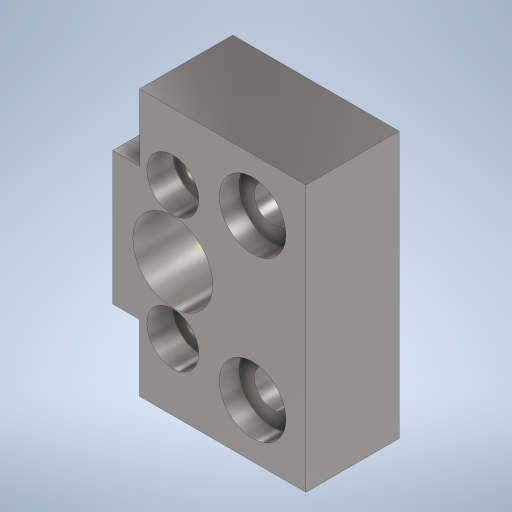
# Autodesk Inventor part: MotorMount
Saved by Autodesk Inventor 2023 (Build 270158000, 158)
## iProperties
Created: 2023-03-27
Part Number: MotorMount
Material: Stainless Steel
Document SubType Name: Modeling
Designer: Nathann
Density: 8 g/cm^3
Appearance: Semi-Polished
Mass: 11.2507 g
Surface Area: 13.5845 cm^2
Volume: 1.40634 cm^3
Author: Nathann
Autodesk Inventor part; units mm, degrees
ref_plane "YZ Plane" through (0, 0, 0) normal (1, 0, 0) x (0, 1, 0)
ref_plane "XZ Plane" through (0, 0, 0) normal (0, 1, 0) x (-1, 0, 0)
ref_plane "XY Plane" through (0, 0, 0) normal (0, 0, 1) x (1, 0, 0)
sketch "Sketch1" plane through (0, 0, 0) normal (0, 0, 1) x (1, 0, 0)
  line L0 (10, -10) -> (-10, -10)
  line L1 (-10, -10) -> (-10, 10)
  line L2 (-10, 10) -> (10, 10)
  line L3 (10, 10) -> (10, -10)
  circle A0 centre (0, 5) radius 1.2
  circle A1 centre (0, -5) radius 1.2
  circle A2 centre (0, 0) radius 3
  dimension "d0" = 10
  dimension "d1" = 10
  dimension "d2" = 10
  dimension "d3" = 10
  dimension "d4" = 5
  dimension "d5" = 5
  dimension "d6" = 2.4
  dimension "d7" = 2.4
  dimension "d8" = 6
  constraints: 8 end point, 3 centre point, 2 parallel, 1 coincident, 1 horizontal, 1 perpendicular
  measures "d0" distance from line of L1 point (0, 0)
  measures "d1" distance from line of L3 point (0, 0)
  measures "d2" distance from line of L0 point (0, 0)
  measures "d3" distance from line of L2 point (0, 0)
  measures "d4" distance of point (0, 0) A0.centre
  measures "d5" distance of point (0, 0) A1.centre
  measures "d6" diameter of A0
  measures "d7" diameter of A1
  measures "d8" diameter of A2
extrude "Extrusion1" add sketch "Sketch1" along normal blind 5
sketch "Sketch2" plane through (0, 0, 5) normal (0, 0, 1) x (1, 0, 0)
  line L0 (0, 0) -> (-1.3346, -1.3533)
  circle A0 centre (6, -6) radius 2.5
  circle A1 centre (6, 6) radius 2.5
  line L1 (10, -10) -> (10, 10) projected
  line L2 (-10, -10) -> (10, -10) projected
  line L3 (10, 10) -> (-10, 10) projected
  dimension "d34" = 4
  dimension "d35" = 4
  dimension "d36" = 4
  dimension "d37" = 4
  dimension "d38" = 5
  dimension "d39" = 5
  constraints: 2 centre point, 2 end point, 1 other
  measures "d34" distance from line of L1 A0.centre
  measures "d35" distance from line of L2 A0.centre
  measures "d36" distance from line of L3 A1.centre
  measures "d37" distance from line of L1 A1.centre
  measures "d38" diameter of A1
  measures "d39" diameter of A0
extrude "Extrusion2" cut sketch "Sketch2" against normal blind 1
sketch "Sketch7" plane through (0, 0, 0) normal (0, 0, -1) x (-1, 0, 0)
  circle A0 centre (-6, 6) radius 2.5 projected
  circle A1 centre (-6, 6) radius 1.375
  circle A2 centre (-6, -6) radius 2.5 projected
  circle A3 centre (-6, -6) radius 1.375
  point P0 (0, 0)
  dimension "d40" = 2.75
  dimension "d41" = 2.75
  constraints: 2 centre point, 2 coincident
  measures "d40" diameter of A1
  measures "d41" diameter of A3
extrude "Extrusion6" cut sketch "Sketch7" against normal blind 5 contours A1 | A3
sketch "Sketch8" plane through (0, 0, 5) normal (0, 0, 1) x (1, 0, 0)
  line L0 (10, 10) -> (-10, 10) projected
  line L1 (10, 10) -> (2.5, 10)
  line L2 (2.5, 10) -> (2.5, 2.5)
  line L3 (2.5, 2.5) -> (10, 2.5)
  line L4 (10, 2.5) -> (10, 10)
  line L5 (10, -10) -> (10, 10) projected
  line L6 (10, -10) -> (2.5, -10)
  line L7 (2.5, -10) -> (2.5, -2.5)
  line L8 (2.5, -2.5) -> (10, -2.5)
  line L9 (10, -2.5) -> (10, -10)
  line L10 (10, -2.5) -> (5, -2.5)
  line L11 (5, -2.5) -> (5, 2.5)
  line L12 (5, 2.5) -> (10, 2.5)
  line L13 (10, 2.5) -> (10, -2.5)
  circle A0 centre (6, 6) radius 2.5 projected
  circle A1 centre (6, 6) radius 2.5
  circle A2 centre (6, -6) radius 2.5 projected
  circle A3 centre (6, -6) radius 2.5
  point P0 (0, 0)
  point P1 (2.5, 10)
  dimension "d44" = 7.5
  dimension "d45" = 7.5
  dimension "d46" = 7.5
  dimension "d47" = 7.5
  dimension "d48" = 5
  constraints: 24 end point, 6 parallel, 3 horizontal, 3 perpendicular, 2 centre point, 2 coincident, 2 point on line
  measures "d44" distance between parallel lines of L4 L2
  measures "d45" distance of L1.end L2.end
  measures "d46" distance of L6.end L7.end
  measures "d47" distance of L5.start L6.end
  measures "d48" distance between parallel lines of L5 L11
extrude "Extrusion7" add sketch "Sketch8" along normal blind 2
sketch "Sketch9" plane through (0, 0, 0) normal (0, 0, -1) x (-1, 0, 0)
  circle A0 centre (-6, 6) radius 1.375 projected
  circle A1 centre (-6, 6) radius 2.5
  circle A2 centre (-6, -6) radius 1.375 projected
  circle A3 centre (-6, -6) radius 2.5
  point P0 (0, 0)
  dimension "d51" = 5
  dimension "d52" = 5
  constraints: 2 centre point, 2 coincident
  measures "d51" diameter of A1
  measures "d52" diameter of A3
extrude "Extrusion8" cut sketch "Sketch9" against normal blind 2.5 contours A0 | A1 | A2 | A3
sketch "Sketch10" plane through (0, 0, 0) normal (0, 0, -1) x (-1, 0, 0)
  line L0 (-2.5, 10) -> (10, 10) projected
  line L1 (10, -10) -> (-2.5, -10) projected
  line L2 (10, 10) -> (5, 10)
  line L3 (5, 10) -> (5, -10)
  line L4 (5, -10) -> (10, -10)
  line L5 (10, -10) -> (10, 10)
  line L6 (5, 10) -> (2.5, 10)
  line L7 (2.5, 10) -> (2.5, 5)
  line L8 (2.5, 5) -> (5, 5)
  line L9 (5, 5) -> (5, 10)
  line L10 (5, -10) -> (2.5, -10)
  line L11 (2.5, -10) -> (2.5, -5)
  line L12 (2.5, -5) -> (5, -5)
  line L13 (5, -5) -> (5, -10)
  point P0 (0, 0)
  point P1 (2.5, 10)
  dimension "d55" = 5
  dimension "d56" = 2.5
  dimension "d57" = 5
  dimension "d58" = 5
  dimension "d59" = 2.5
  constraints: 24 end point, 6 parallel, 3 horizontal, 3 perpendicular, 2 point on line
  measures "d55" distance between parallel lines of L5 L3
  measures "d56" distance of L7.end L8.end
  measures "d57" distance of L6.end L7.end
  measures "d58" distance of L10.end L11.end
  measures "d59" distance of L11.end L12.end
extrude "Extrusion9" cut sketch "Sketch10" against normal blind 10
sketch "Sketch12" plane through (6, -6, 4) normal (0, 0, 1) x (1, 0, 0)
  circle A0 centre (0, 0) radius 1.375 projected
  circle A1 centre (0, 0) radius 2.5 projected
  circle A2 centre (0, 12) radius 2.5 projected
  circle A3 centre (0, 12) radius 1.375 projected
  circle A4 centre (0, 12) radius 2.5 projected
  point P0 (-6, 6)
extrude "Extrusion11" add sketch "Sketch12" along normal blind 1.5
sketch "Sketch13" plane through (0, 0, 5) normal (0, 0, 1) x (1, 0, 0)
  point P0 (0, 0)
sketch "Sketch14" plane through (0, 0, 5) normal (0, 0, 1) x (1, 0, 0)
  line L0 (-2.5, -5) -> (-2.5, -10) projected
  line L1 (-2.5, -10) -> (2.5, -10) projected
  line L2 (2.5, -10) -> (2.5, -2.5) projected
  line L3 (2.5, -2.5) -> (5, -2.5) projected
  line L4 (5, -2.5) -> (5, 2.5) projected
  line L5 (5, 2.5) -> (2.5, 2.5) projected
  line L6 (2.5, 2.5) -> (2.5, 10) projected
  line L7 (2.5, 10) -> (-2.5, 10) projected
  line L8 (-2.5, 10) -> (-2.5, 5) projected
  line L9 (-2.5, 5) -> (-5, 5) projected
  line L10 (-5, 5) -> (-5, -5) projected
  line L11 (-5, -5) -> (-2.5, -5) projected
  circle A0 centre (0, 0) radius 3 projected
  circle A1 centre (0, -5) radius 1.2 projected
  circle A2 centre (0, 5) radius 1.2 projected
  circle A3 centre (0, -5) radius 1.95
  circle A4 centre (0, 5) radius 1.95
  dimension "d80" = 3.9
  dimension "d81" = 3.9
  constraints: 2 centre point, 2 coincident
  measures "d80" diameter of A3
  measures "d81" diameter of A4
extrude "Extrusion12" add sketch "Sketch14" along normal blind 2 contours L11 L10 L9 L8 L7 L6 L5 L4 L3 L2 L1 L0
sketch "Sketch15" plane through (-5, -5, 0) normal (-1, 0, 0) x (0, 0, 1)
  line L0 (0, 10) -> (7, 10) projected
  line L1 (0, 0) -> (0, 10) projected
  line L2 (0, 0) -> (7, 0) projected
  line L3 (7, 10) -> (7, 0) projected
  point P0 (0, 5)
extrude "Extrusion13" cut sketch "Sketch15" against normal blind 0.5
equation "\"d1\" = d0"
equation "\"d2\" = d0"
equation "\"d3\" = d2"
equation "\"d5\" = d4"
equation "\"d7\" = d6"
equation "\"d39\" = d38"
equation "\"d45\" = d44"
equation "\"d46\" = d45"
equation "\"d52\" = d51"
equation "\"d81\" = d80"
body "Solid1"
